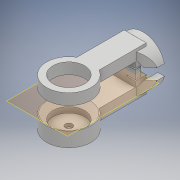
# Autodesk Inventor part: baseRotor1
Saved by Autodesk Inventor 2017 (Build 210142000, 142)
## iProperties
Created: 2017-08-06
Part Number: baseRotor1
Material: Generic
Document SubType Name: Sheet Metal
Designer: Bardo91
Density: 1 g/cm^3
Sheet Metal Rule: Default_mm
Appearance: Default
Author: Bardo91
Autodesk Inventor part; units mm, degrees
ref_plane "YZ Plane" through (0, 0, 0) normal (1, 0, 0) x (0, 1, 0)
ref_plane "XZ Plane" through (0, 0, 0) normal (0, 1, 0) x (-1, 0, 0)
ref_plane "XY Plane" through (0, 0, 0) normal (0, 0, 1) x (1, 0, 0)
sketch "Sketch1" plane through (0, 0, 0) normal (0, 0, 1) x (1, 0, 0)
  circle A0 centre (0, 0) radius 14.25
  circle A1 centre (0, 0) radius 20
  line L0 (0, 50) -> (10, 50)
  line L1 (10, 50) -> (10, 17.3205)
  line L2 (0, 20) -> (0, 50)
  line L3 (0, 50) -> (-10, 50)
  line L4 (-10, 50) -> (-10, 17.3205)
  point P0 (-20, 0)
  point P1 (20, 0)
  dimension "d0" = 28.5
  dimension "d1" = 40
  dimension "d25" = 10
  dimension "d31" = 10
  constraints: 10 end point, 5 point on circle, 2 centre point, 2 coincident, 2 perpendicular, 1 horizontal
  measures "d0" diameter of A0
  measures "d1" diameter of A1
  measures "d25" distance of L0.end L0.start
  measures "d31" distance of L0.start L3.end
extrude "Extrusion1" add sketch "Sketch1" along normal blind 10
ref_plane "Work Plane1" through (0, 0, -10) normal (0, 0, 1) x (1, 0, 0)
mirror "Mirror1" about plane through (0, 0, -10) normal (0, 0, 1) of "Extrusion1"
sketch "Sketch2" plane through (0, 0, -30) normal (0, 0, -1) x (-1, 0, 0)
  circle A0 centre (0, 0) radius 14.25 projected
  circle A1 centre (0, 0) radius 20
  dimension "d11" = 40
  constraints: 1 centre point, 1 coincident
  measures "d11" diameter of A1
extrude "Extrusion2" add sketch "Sketch2" along normal blind 3 contours A0 | A1
sketch "Sketch3" plane through (0, 0, -30) normal (0, 0, 1) x (1, 0, 0)
  circle A0 centre (0, 0) radius 3.15
  dimension "d14" = 6.3
  constraints: 1 centre point, 1 coincident
  measures "d14" diameter of A0
extrude "Extrusion3" cut sketch "Sketch3" against normal blind 1
sketch "Sketch4" plane through (0, 0, -31) normal (0, 0, 1) x (1, 0, 0)
  circle A0 centre (0, 0) radius 3.15
  line L0 (0, 0) -> (0, -1.6)
  line L1 (0, -1.6) -> (-2.7134, -1.6)
  line L2 (0, -1.6) -> (2.7134, -1.6)
  dimension "d17" = 6.3
  dimension "d18" = 1.6
  constraints: 6 end point, 2 horizontal, 2 point on circle, 1 centre point, 1 coincident, 1 vertical
  measures "d17" diameter of A0
  measures "d18" distance of L0.start L0.end
extrude "Extrusion4" cut sketch "Sketch4" against normal through all contours A0 L2 L1 picked at (-0.0447, 1.5505)
sketch "Sketch6" plane through (-7.5, 50, -22) normal (0, 1, 0) x (1, 0, 0)
  line L0 (17.5, 8) -> (17.5, 8) projected
  line L1 (17.5, -22) -> (17.5, -32) projected
  line L2 (-2.5, 8) -> (17.5, 8)
  line L3 (17.5, 8) -> (17.5, -32)
  line L4 (17.5, -32) -> (-2.5, -32)
  line L5 (-2.5, -32) -> (-2.5, 8)
  point P0 (7.5, -22)
  constraints: 8 end point, 2 parallel, 1 horizontal, 1 horizontal alignment, 1 perpendicular
extrude "Extrusion6" add sketch "Sketch6" along normal blind 10
chamfer "Chamfer1" distance 5 angle 45 1 edges at (-14.25, 0, -20)
sketch "Sketch9" plane through (-7.5, 60, -22) normal (0, 1, 0) x (1, 0, 0)
  line L0 (-2.5, 8) -> (-2.5, -32) projected
  line L1 (-2.5, -32) -> (17.5, -32)
  line L2 (-2.5, -32) -> (17.5, -32) projected
  line L3 (7.5, -32) -> (7.5, -12)
  line L4 (7.5, -12) -> (1.75, -12)
  line L5 (1.75, -12) -> (1.75, -17)
  line L6 (1.75, -17) -> (21.75, -17)
  line L7 (21.75, -17) -> (21.75, -7)
  line L8 (21.75, -7) -> (1.75, -7)
  line L9 (1.75, -7) -> (1.75, -12)
  point P0 (7.5, -22)
  dimension "d38" = 20
  dimension "d39" = 5.75
  dimension "d40" = 5
  dimension "d41" = 20
  dimension "d42" = 10
  constraints: 16 end point, 5 perpendicular, 2 horizontal, 1 midpoint, 1 point on line, 1 vertical
  measures "d38" distance of L3.start L3.end
  measures "d39" distance of L3.end L4.end
  measures "d40" distance of L4.end L5.end
  measures "d41" distance of L5.end L6.end
  measures "d42" distance of L6.end L7.end
extrude "Extrusion9" cut sketch "Sketch9" against normal blind 5
sketch "Sketch10" plane through (-7.5, 55, -22) normal (0, 1, 0) x (1, 0, 0)
  line L0 (1.75, -17) -> (1.75, -7) projected
  line L1 (1.75, -17) -> (9.75, -17)
  line L2 (17.5, -17) -> (1.75, -17) projected
  line L3 (9.75, -17) -> (9.75, -16)
  line L4 (9.75, -16) -> (17.5, -16)
  line L5 (17.5, -16) -> (17.5, -17)
  line L6 (17.5, -17) -> (9.75, -17)
  line L7 (1.75, -7) -> (17.5, -7) projected
  line L8 (1.75, -7) -> (9.75, -7)
  line L9 (9.75, -7) -> (9.75, -8)
  line L10 (9.75, -8) -> (17.5, -8)
  line L11 (17.5, -8) -> (17.5, -7)
  line L12 (17.5, -2) -> (17.5, -22) projected
  line L13 (9.75, -7) -> (17.5, -7)
  point P0 (7.5, -22)
  dimension "d45" = 8
  dimension "d46" = 1
  dimension "d47" = 90
  dimension "d48" = 8
  dimension "d49" = 1
  constraints: 20 end point, 6 point on line, 5 perpendicular, 1 parallel
  measures "d45" distance of L0.start L1.end
  measures "d46" distance of L1.end L3.end
  measures "d47" angle of L3 L1
  measures "d48" distance of L0.end L8.end
  measures "d49" distance of L8.end L9.end
extrude "Extrusion10" cut sketch "Sketch10" against normal blind 5 contours L3 L4 L5 L2 | L7 L11 L10 L9
sketch "Sketch11" plane through (-7.5, 60, -22) normal (0, 1, 0) x (1, 0, 0)
  line L0 (-2.5, -32) -> (17.5, -32) projected
  line L1 (7.5, -32) -> (7.5, -12)
  circle A0 centre (7.5, -12) radius 14.25
  circle A1 centre (7.5, -12) radius 20
  point P0 (7.5, -22)
  dimension "d52" = 20
  dimension "d53" = 28.5
  dimension "d54" = 40
  constraints: 2 centre point, 2 coincident, 2 end point, 1 midpoint, 1 vertical
  measures "d52" distance of L1.start L1.end
  measures "d53" diameter of A0
  measures "d54" diameter of A1
extrude "Extrusion11" add sketch "Sketch11" along normal blind 7
sketch "Sketch12" plane through (0, 67, -10) normal (0, 1, 0) x (1, 0, 0)
  line L0 (0, 0) -> (0, -5)
  line L1 (0, -5) -> (25, -5)
  line L2 (0, 0) -> (0, 5)
  line L3 (0, 5) -> (25, 5)
  line L4 (25, 5) -> (25, -5)
  point P0 (0, -10)
  dimension "d57" = 5
  dimension "d58" = 25
  dimension "d59" = 5
  dimension "d60" = 25
  constraints: 10 end point, 2 perpendicular, 1 point on line, 1 vertical
  measures "d57" distance of L0.start L0.end
  measures "d58" distance of L0.end L1.end
  measures "d59" distance of L0.start L2.end
  measures "d60" distance of L2.end L3.end
extrude "Extrusion12" cut sketch "Sketch12" against normal up to surface (7 mm away)
chamfer "Chamfer2" distance 9 angle 45 2 edges at (10, 60, -23.7362) (10, 60, 3.7362)
chamfer "Chamfer3" distance 4 angle 45 2 edges at (-10, 60, 3.7362) (-10, 60, -23.7362)
sketch "Sketch13" plane through (-7.5, 55, -22) normal (0, 1, 0) x (1, 0, 0)
  line L0 (1.75, -17) -> (1.75, -7) projected
  line L1 (1.75, -7) -> (1.75, -9)
  line L2 (1.75, -9) -> (3.05, -9)
  line L3 (3.05, -9) -> (3.05, -15)
  line L4 (3.05, -9) -> (3.05, -12)
  line L5 (3.05, -9) -> (11.45, -9)
  line L6 (11.45, -9) -> (11.45, -12)
  line L7 (11.45, -12) -> (11.45, -15)
  circle A0 centre (11.45, -9) radius 0.9
  circle A1 centre (11.45, -15) radius 0.9
  circle A2 centre (11.45, -12) radius 0.9
  circle A3 centre (3.05, -9) radius 0.9
  circle A4 centre (3.05, -12) radius 0.9
  circle A5 centre (3.05, -15) radius 0.9
  point P0 (7.5, -22)
  dimension "d69" = 2
  dimension "d70" = 1.3
  dimension "d71" = 6
  dimension "d72" = 3
  dimension "d73" = 8.4
  dimension "d74" = 3
  dimension "d75" = 3
  dimension "d76" = 1.8
  dimension "d77" = 1.8
  dimension "d78" = 1.8
  dimension "d79" = 1.8
  dimension "d80" = 1.8
  dimension "d81" = 1.8
  constraints: 14 end point, 6 centre point, 6 coincident, 3 perpendicular, 2 point on line, 1 horizontal, 1 midpoint
  measures "d69" distance of L0.end L1.end
  measures "d70" distance of L1.end L2.end
  measures "d71" distance of L2.end L3.end
  measures "d72" distance of L2.end L4.end
  measures "d73" distance of L2.end L5.end
  measures "d74" distance of L5.end L6.end
  measures "d75" distance of L6.end L7.end
  measures "d76" diameter of A0
  measures "d77" diameter of A1
  measures "d78" diameter of A2
  measures "d79" diameter of A3
  measures "d80" diameter of A4
  measures "d81" diameter of A5
extrude "Extrusion13" cut sketch "Sketch13" against normal blind 2.5
equation "\"d4\" = d25"
equation "\"d76\" = d78"
equation "\"d78\" = d77"
equation "\"d79\" = d77"
equation "\"d80\" = d77"
equation "\"d81\" = d77"
equation "\"BendRadius\" = Thickness"
equation "\"BendReliefWidth\" = Thickness"
equation "\"BendReliefDepth\" = 0.5 * Thickness"
equation "\"CornerReliefSize\" = 4 * Thickness"
equation "\"MinimumRemnant\" = 2 * Thickness"
equation "\"TransitionRadius\" = BendRadius"
equation "\"JacobiRadiusSize\" = BendRadius"
equation "\"GapSize\" = Thickness"
equation "\"Thickness\" = 0.5"
body "Solid1"
